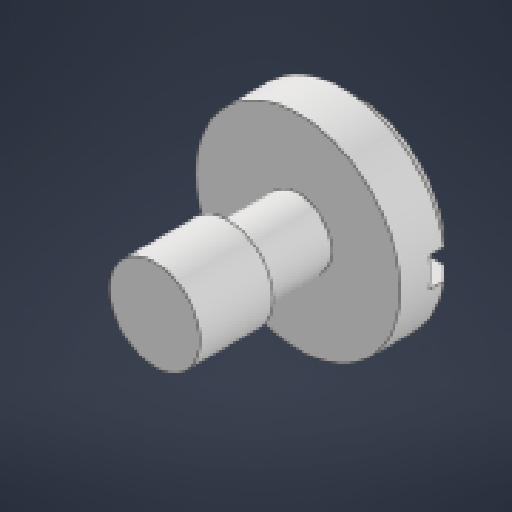
# Autodesk Inventor part: AccessoryScrew
Saved by Autodesk Inventor 2023 (Build 270158000, 158)
## iProperties
Created: 2023-02-18
Part Number: AccessoryScrew
Material: Generic
Document SubType Name: Modeling
Designer: jevan
Density: 1 g/cm^3
Appearance: Default
Author: jevan
Autodesk Inventor part; units mm, degrees
ref_plane "YZ Plane" through (0, 0, 0) normal (1, 0, 0) x (0, 1, 0)
ref_plane "XZ Plane" through (0, 0, 0) normal (0, 1, 0) x (-1, 0, 0)
ref_plane "XY Plane" through (0, 0, 0) normal (0, 0, 1) x (1, 0, 0)
sketch "Sketch1" plane through (0, 0, 0) normal (0, 0, 1) x (1, 0, 0)
  circle A0 centre (0, 0) radius 7
  circle A1 centre (0, 0) radius 2.3
  circle A2 centre (0, 0) radius 3.11
  dimension "d0" = 14
  dimension "d1" = 4.6
  dimension "d2" = 6.22
  constraints: 3 centre point, 3 coincident
  measures "d0" diameter of A0
  measures "d1" diameter of A1
  measures "d2" diameter of A2
extrude "Extrusion1" add sketch "Sketch1" against normal blind 4.06 contours A0 | A1 | A2
extrude "Extrusion2" add sketch "Sketch1" along normal blind 9.82 contours A1 | A2
extrude "Extrusion3" cut sketch "Sketch1" along normal blind 4.82 contours A2
sketch "Sketch2" plane through (0, 0, -4.06) normal (0, 0, -1) x (-1, 0, 0)
  line L0 (7, 1) -> (-7, 1)
  line L1 (-7, 1) -> (-7, -1)
  line L2 (-7, -1) -> (7, -1)
  line L3 (7, -1) -> (7, 1)
  line L4 (7, 1) -> (-7, -1) construction
  line L5 (-7, 1) -> (7, -1) construction
  point P0 (0, 0)
  dimension "d9" = 2
  constraints: 12 end point, 2 midpoint, 2 parallel, 1 horizontal, 1 perpendicular
  measures "d9" distance of L1.end L0.end
extrude "Extrusion4" cut sketch "Sketch2" against normal blind 2
chamfer "Chamfer1" distance 1 angle 45 2 edges at (0, -7, -4.06) (0, 7, -4.06)
body "Solid1"
